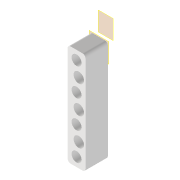
# Autodesk Inventor part: Omniscope_USBC_Bar_lenses
Saved by Autodesk Inventor 2022 (Build 260153000, 153)
## iProperties
Created: 2023-05-17
Part Number: Omniscope_USBC_Bar_lenses
Material: Generisch
Document SubType Name: Modeling
Designer: diederichbenedict
Density: 1 g/cm^3
Appearance: Vorgabe
Author: diederichbenedict
Autodesk Inventor part; units mm, degrees
ref_plane "YZ Plane" through (0, 0, 0) normal (1, 0, 0) x (0, 1, 0)
ref_plane "XZ Plane" through (0, 0, 0) normal (0, 1, 0) x (-1, 0, 0)
ref_plane "XY Plane" through (0, 0, 0) normal (0, 0, 1) x (1, 0, 0)
ref_plane "Arbeitsebene1" through (0, 0, 0) normal (0, 0, 1) x (1, 0, 0)
ref_plane "Arbeitsebene2" through (-1.5, 28.05, 3) normal (0, 0, 1) x (0, -1, 0)
sketch "Skizze2" plane through (-1.5, 28.05, 3) normal (0, 0, 1) x (0, -1, 0)
  circle A0 centre (56.1, 0) radius 4 construction
  circle A1 centre (56.1, 0) radius 3.65
  circle A2 centre (37.4, 0) radius 4 construction
  circle A3 centre (18.7, 0) radius 4 construction
  line L0 (6.2, -3) -> (-6.2, -3) construction
  circle A4 centre (0, 0) radius 4 construction
  circle A5 centre (37.4, 0) radius 3.6
  circle A6 centre (18.7, 0) radius 3.6
  circle A7 centre (0, 0) radius 3.6
  circle A8 centre (66, 1.5) radius 1.4 construction
  circle A9 centre (46.75, 1.5) radius 1.4 construction
  circle A10 centre (28.05, 1.5) radius 1.4 construction
  circle A11 centre (9.35, 1.5) radius 1.4 construction
  circle A12 centre (-9.9, 1.5) radius 1.4 construction
  circle A13 centre (66, 1.5) radius 1.6
  circle A14 centre (46.75, 1.5) radius 1.6
  circle A15 centre (28.05, 1.5) radius 1.6
  circle A16 centre (9.35, 1.5) radius 1.6
  circle A17 centre (-9.9, 1.5) radius 1.6
  line L1 (6, 6) -> (6, -6) projected
  line L2 (-6, 6) -> (6, 6) projected
  line L3 (-6, -6) -> (-6, 6) projected
  line L4 (6, -6) -> (-6, -6) projected
  circle A18 centre (0, 0) radius 4 projected
  line L5 (62.1, 6) -> (62.1, -6) projected
  line L6 (50.1, 6) -> (62.1, 6) projected
  line L7 (50.1, -6) -> (50.1, 6) projected
  line L8 (62.1, -6) -> (50.1, -6) projected
  circle A19 centre (56.1, 0) radius 4 projected
  line L9 (69.1, 6) -> (-12.4207, 6)
  line L10 (-12.4207, 6) -> (-12.4207, -6)
  line L11 (-12.4207, -6) -> (69.1, -6)
  line L12 (69.1, -6) -> (69.1, 6)
  point P0 (28.05, 1.5)
  point P1 (50.1, 6)
  point P2 (6, 6)
  point P3 (6, -6)
  dimension "d0" = 7.3
  dimension "d1" = 7.2
  dimension "d2" = 7.2
  dimension "d3" = 7.2
  dimension "d4" = 3.2
  dimension "d5" = 3.2
  dimension "d6" = 3.2
  dimension "d7" = 3.2
  dimension "d8" = 3.2
  dimension "d9" = 7
  constraints: 9 centre point, 9 coincident, 8 end point, 2 parallel, 1 horizontal, 1 perpendicular, 2 other
  measures "d0" diameter of A1
  measures "d1" diameter of A5
  measures "d2" diameter of A6
  measures "d3" diameter of A7
  measures "d4" diameter of A13
  measures "d5" diameter of A14
  measures "d6" diameter of A15
  measures "d7" diameter of A16
  measures "d8" diameter of A17
  measures "d9" distance from line of L12 L5.start
extrude "Extrusion1" add sketch "Skizze2" along normal blind 10 contours L9 L7 L11 L1 | L1 L4 L3 L2 | L6 L5 L8 L7 | A18 | A19
sketch "Skizze3" plane through (-1.5, 28.05, 13) normal (0, 0, 1) x (1, 0, 0)
  line L0 (-6, 6) -> (-6, -62.1) projected
  line L1 (-6, -62.1) -> (6, -62.1) projected
  line L2 (6, -62.1) -> (6, 6) projected
  line L3 (6, 6) -> (-6, 6) projected
  circle A0 centre (1.5, -9.35) radius 1.6 projected
  circle A1 centre (1.5, -28.05) radius 1.6 projected
  circle A2 centre (1.5, -46.75) radius 1.6 projected
  circle A3 centre (0, -18.7) radius 3.6 projected
  circle A4 centre (0, -37.4) radius 3.6 projected
  circle A5 centre (0, 0) radius 3.6 projected
  circle A6 centre (0, -56.1) radius 3.35
  circle A7 centre (0, -37.4) radius 3.6 projected
  circle A8 centre (0, -37.4) radius 3.35
  circle A9 centre (0, -18.7) radius 3.6 projected
  circle A10 centre (0, -18.7) radius 3.35
  circle A11 centre (0, 0) radius 3.35
  point P0 (1.5, -28.05)
  dimension "d12" = 6.7
  dimension "d13" = 6.7
  dimension "d14" = 6.7
  dimension "d15" = 6.7
  constraints: 4 centre point, 3 coincident
  measures "d12" diameter of A6
  measures "d13" diameter of A8
  measures "d14" diameter of A10
  measures "d15" diameter of A11
extrude "Extrusion2" add sketch "Skizze3" along normal blind 5 contours L3 L2 L1 L0 | A3 | A4 | A5
sketch "Skizze4" plane through (-1.5, 28.05, 18) normal (0, 0, 1) x (1, 0, 0)
  circle A0 centre (1.5, -46.75) radius 1.6 projected
  circle A1 centre (1.5, -28.05) radius 1.6 projected
  circle A2 centre (1.5, -9.35) radius 1.6 projected
  point P0 (1.5, -28.05)
hole "Bohrung1" at (0, -18.7, 18) at (0, 0, 18) at (0, 18.7, 18) direction (0, 0, -1) diameter 3.2 end through all counterbore diameter 7 counterbore depth 10
fillet "Rundung1" radius 2 4 edges at (4.5, -34.05, 10.5) (-7.5, -34.05, 10.5) (-7.5, 34.05, 10.5) (4.5, 34.05, 10.5)
